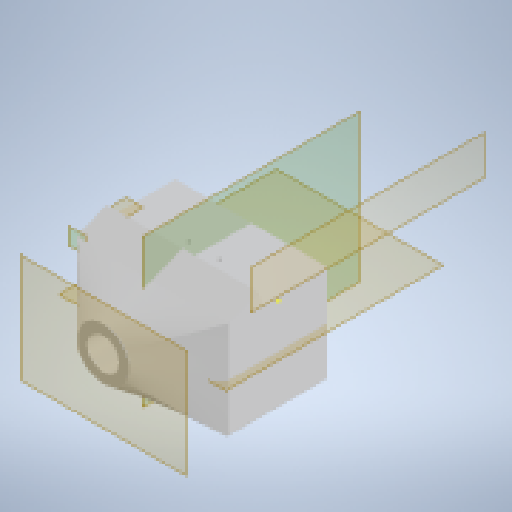
# Autodesk Inventor part: WingBoxCouple
Saved by Autodesk Inventor 2026 (Build 300175050, 175E)
## iProperties
Created: 2025-07-20
Part Number: WingBoxCouple
Material: Generic
Document SubType Name: Modeling
Designer: Cupri
Density: 1 g/cm^3
Appearance: Default
Author: Cupri
Autodesk Inventor part; units mm, degrees
ref_plane "YZ Plane" through (0, 0, 0) normal (1, 0, 0) x (0, 1, 0)
ref_plane "XZ Plane" through (0, 0, 0) normal (0, 1, 0) x (-1, 0, 0)
ref_plane "Work Plane9" through (-195, -6.556, 63.7436) normal (0, 0, -1) x (-1, 0, 0)
sketch "Sketch8" plane through (-195, -6.556, 63.7436) normal (0, 0, -1) x (-1, 0, 0)
  line L0 (0, 4.9685) -> (-195, 4.9685) projected
  line L1 (0, 4.9685) -> (-195, 4.9685)
  line L2 (-195, 4.9685) -> (-195, -122.0315)
  line L3 (-195, -122.0315) -> (0, -122.0315)
  line L4 (0, -122.0315) -> (0, 4.9685)
  line L5 (-6.35, -1.3815) -> (-188.65, -1.3815)
  line L6 (-188.65, -1.3815) -> (-188.65, -115.6815)
  line L7 (-188.65, -115.6815) -> (-6.35, -115.6815)
  line L8 (-6.35, -115.6815) -> (-6.35, -1.3815)
  point P0 (-195, 6.556)
  dimension "d11" = 127
  dimension "d12" = 6.35
  dimension "d13" = 6.35
  dimension "d14" = 6.35
  dimension "d15" = 6.35
  constraints: 16 end point, 4 parallel, 2 horizontal, 2 perpendicular
  measures "d11" distance of L2.end L1.end
  measures "d12" distance between parallel lines of L2 L6
  measures "d13" distance between parallel lines of L0 L5
  measures "d14" distance between parallel lines of L3 L7
  measures "d15" distance between parallel lines of L4 L8
extrude "Extrusion4" add sketch "Sketch8" along normal blind 127
ref_plane "Work Plane8" through (-195, -1.5875, 0) normal (0, 1, 0) x (1, 0, 0)
ref_plane "Work Plane2" through (-97.5, 44.244, 0) normal (-1, 0, 0) x (0, 0, 1)
ref_plane "Work Plane3" through (0, -65.0875, 0) normal (0, 1, 0) x (1, 0, 0)
ref_plane "Work Plane11" through (-195, -6.556, 127.2436) normal (0, 0, 1) x (1, 0, 0)
sketch "Sketch12" plane through (-195, -6.556, 127.2436) normal (0, 0, 1) x (1, 0, 0)
  line L0 (0, -122.0315) -> (0, 4.9685) projected
  line L1 (0, -45.8315) -> (195, -45.8315) construction
  line L2 (195, 4.9685) -> (195, -122.0315) projected
  line L3 (195, -122.0315) -> (0, -122.0315) projected
  circle A0 centre (97.5, -45.8315) radius 20.447
  circle A1 centre (97.5, -45.8315) radius 33.147
  point P0 (195, 6.556)
  dimension "d35" = 76.2
  dimension "d36" = 40.894
  dimension "d38" = 12.7
  constraints: 2 centre point, 2 end point, 2 point on line, 1 coincident, 1 horizontal, 1 midpoint
  measures "d35" distance between parallel lines of L3 L1
  measures "d36" diameter of A0
  measures "d38" radial gap between concentric circles of A0 A1
loft "Loft1" add profiles "Sketch12" section 2 edges at (-97.5, -1.5875, 63.7436) (-195, -65.0875, 63.7436) (-97.5, -128.5875, 63.7436) (0, -65.0875, 63.7436) contours A0 | A1
sketch "Sketch13" plane through (-97.5, -52.3875, 127.2436) normal (0, 0, 1) x (1, 0, 0)
  circle A0 centre (0, 0) radius 20.447
  point P0 (97.5, 52.3875)
  dimension "d45" = 40.894
  constraints: 1 centre point
  measures "d45" diameter of A0
extrude "Extrusion8" cut sketch "Sketch13" against normal blind 127
ref_plane "Work Plane12" through (-0.0207, 21.3282, -116.2129) normal (1, 0, 0) x (0, 0, -1)
sketch "Sketch15" plane through (0, -128.5875, -63.2564) normal (1, 0, 0) x (0, 0, -1)
  line L0 (-84.3534, 127) -> (-84.3534, 143.7527)
  line L1 (-127, 127) -> (-127, 0) projected
  line L2 (-127, 127) -> (-85.2319, 144.3391)
  line L3 (-127, 127) -> (0, 127) projected
  line L4 (-84.3534, 127) -> (-127, 127)
  line L5 (-85.2319, 144.3391) -> (-84.3534, 144.7038)
  line L6 (-84.3534, 143.7527) -> (-84.3534, 144.7038)
  point P0 (-63.2564, 128.5875)
  dimension "d48" = 17.7038
  dimension "d49" = 42.6466
  constraints: 10 end point, 2 point on line, 2 vertical, 1 perpendicular
  measures "d48" distance of L0.start L5.end
  measures "d49" distance between parallel lines of L0 L1
extrude "Extrusion9" add sketch "Sketch15" against normal up to surface (195 mm away)
chamfer "Chamfer2" distance 4.7625 distance2 15.875 1 edges at (-97.5, 16.1163, 21.097) measured on face at (-97.5, 15.9246, 21.5588)
ref_plane "Work Plane13" through (-195.0366, -1.5723, -251.9517) normal (0, -1, 0) x (1, 0, 0)
fillet "Fillet3" radius 3.175 2 edges at (-195, -128.5875, 0.2436) (0, -128.5875, 0.2436)
body "Solid1"
